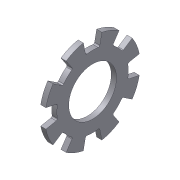
# Autodesk Inventor part: ASME B18.21.1 - 1/4. Carbon Steel
Saved by Autodesk Inventor 2012 SP1 (Build 160190100, 190)
## iProperties
Library Location: D:\Program Files\Autodesk\Inventor 6\content
Library: local
SubLibrary: ANSI
Family: 1059
Member: 80
Member Major Revision: 1
Member Minor Revision: 1
Comments: To add or edit properties for Autodesk Inventor files, use iProperties.
Created: 2003-01-12
Part Number: ASME B18.21.1 - 1/4. Carbon Steel
Vendor: Autodesk Inc.
Document SubType Name: Modeling
Designer: geyerm
Description: External Tooth Lock Washer Type A
Standard: ASME B18.21.1 1/4. Carbon Steel
Material: Steel, Mild
Density: 7.86 g/cm^3
Alert: To add or edit properties for Autodesk Inventor files, use iProperties.
Control State: 0
Master: False
Checked Out: False
Shininess: 64.0
Length Units: 11269
Angle Units: 11279
Time Units: 11290
Mass Units: 11283
Length Display Precision: 3
Angle Display Precision: 2
Classification: un/spsc 31161801
Density: 0.0
Volumn: 0.0
Area: 0.0
PropertySet Name: Model Information
Author: Autodesk
Revision Number: 1
Autodesk Inventor part; units mm, degrees
ref_plane "YZ Plane" through (0, 0, 0) normal (1, 0, 0) x (0, 1, 0)
ref_plane "XZ Plane" through (0, 0, 0) normal (0, 1, 0) x (-1, 0, 0)
ref_plane "XY Plane" through (0, 0, 0) normal (0, 0, 1) x (1, 0, 0)
sketch "Sketch1" plane through (0, 0, 0) normal (1, 0, 0) x (0, 1, 0)
  circle A0 centre (0, 0) radius 6.477
  circle A1 centre (0, 0) radius 3.2512
  dimension "d0" = 12.954
  dimension "d1" = 6.5024
  constraints: 2 centre point, 1 coincident, 1 other
  measures "d0" diameter of A0
  measures "d1" diameter of A1
extrude "Body" add sketch "Sketch1" along normal blind 0.7112
sketch "Sketch2" plane through (0.7112, 0, 0) normal (1, 0, 0) x (0, 0, -1)
  circle A0 centre (0, 0) radius 6.477 projected
  line L0 (0, 0) -> (0, 6.477) construction
  arc A1 (1.2636, 6.3525) -> (-1.2636, 6.3525) centre (0, 0) ccw
  arc A2 (0.9489, 4.7706) -> (-0.9489, 4.7706) centre (0, 0) ccw
  line L1 (-0.9489, 4.7706) -> (-1.2636, 6.3525)
  line L2 (0.9489, 4.7706) -> (1.2636, 6.3525)
  line L3 (-0.9489, 4.7706) -> (0, 0) construction
  line L4 (0, 0) -> (0.9489, 4.7706) construction
  dimension "d4" = 22.5
  dimension "d5" = 9.7282
  constraints: 10 end point, 7 point on circle, 2 centre point, 2 coincident, 2 collinear, 1 concentric, 1 symmetric about line, 1 vertical
  measures "d4" angle of L2 L1
  measures "d5" diameter of A2
extrude "Cut" cut sketch "Sketch2" against normal through all contours L2 A2 L1 A0 picked at (-0.106, 5.9266)
fillet "Fillet1" radius 0.1943 2 edges at (0.3556, 4.7706, 0.9489) (0.3556, 4.7706, -0.9489)
pattern_circular "Cuts" count 8 over 360 about axis through (0, 0, 0) along (1, 0, 0) of "Cut", "Fillet1"
equation "\"d0\" = SD2"
equation "\"d1\" = SD1"
equation "\"d2\" = SD"
equation "\"d5\" = 0.5 * SD2 + 0.5 * SD1"
equation "\"d6\" = SD"
equation "\"d8\" = 0.015 * SD2"
equation "\"SD\" = 0.7112"
equation "\"SD1\" = 6.5024"
equation "\"SD2\" = 12.954"
equation "\"NND\" = 6.35"
body "Solid1"
